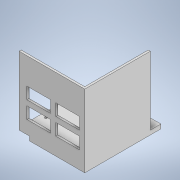
# Autodesk Inventor part: QUarter1
Saved by Autodesk Inventor 2020.2 (Build 242310000, 310)
## iProperties
Created: 2020-01-16
Part Number: QUarter1
Material: Generic
Document SubType Name: Modeling
Designer: ColinP
Density: 1 g/cm^3
Appearance: Default
Author: ColinP
Autodesk Inventor part; units mm, degrees
ref_plane "YZ Plane" through (0, 0, 0) normal (1, 0, 0) x (0, 1, 0)
ref_plane "XZ Plane" through (0, 0, 0) normal (0, 1, 0) x (-1, 0, 0)
ref_plane "XY Plane" through (0, 0, 0) normal (0, 0, 1) x (1, 0, 0)
sketch "Sketch3" plane through (0, 0, 0) normal (0, 1, 0) x (-1, 0, 0)
  line L0 (0, 0) -> (125, 0)
  line L1 (125, 0) -> (125, 125)
  line L2 (125, 125) -> (0, 125)
  line L3 (0, 125) -> (0, 0)
  dimension "d10" = 125
  dimension "d11" = 125
  constraints: 8 end point, 2 parallel, 1 horizontal, 1 perpendicular
  measures "d10" distance of L2.end L1.end
  measures "d11" distance of L1.end L0.end
extrude "Extrusion3" add sketch "Sketch3" along normal blind 10
sketch "Sketch8" plane through (0, 10, 0) normal (0, 1, 0) x (1, 0, 0)
  line L0 (0, 0) -> (-125, 0) projected
  line L1 (0, 0) -> (-4, 0)
  line L2 (-4, 0) -> (-4, -121)
  line L3 (-125, -125) -> (0, -125) projected
  line L4 (-4, -121) -> (-125, -121)
  line L5 (-125, 0) -> (-125, -125) projected
  line L6 (0, 0) -> (-125, 0) projected
  line L7 (-125, 0) -> (-125, -125) projected
  line L8 (-125, -125) -> (0, -125) projected
  line L9 (0, -125) -> (0, 0) projected
  dimension "d38" = 4
  dimension "d39" = 121
  dimension "d40" = 90
  constraints: 6 end point, 2 point on line, 1 perpendicular
  measures "d38" distance of L0.start L1.end
  measures "d39" distance of L1.end L2.end
  measures "d40" angle of L2 L4
extrude "Extrusion8" add sketch "Sketch8" along normal blind 125 contours L9 L3 L5 L4 L2 L0
sketch "Sketch9" plane through (-125, 0, 125) normal (0, 0, 1) x (1, 0, 0)
  line L0 (0, 0) -> (0, 10) projected
  line L1 (0, 10) -> (0, 30)
  line L2 (0, 0) -> (0, 135) projected
  line L3 (0, 30) -> (15, 30)
  line L4 (15, 30) -> (60, 30)
  line L5 (60, 30) -> (60, 52.5)
  line L6 (60, 52.5) -> (15, 52.5)
  line L7 (15, 52.5) -> (15, 30)
  line L8 (15, 52.5) -> (15, 62.5)
  line L9 (15, 62.5) -> (15, 85)
  line L10 (15, 85) -> (60, 85)
  line L11 (60, 85) -> (60, 62.5)
  line L12 (60, 62.5) -> (15, 62.5)
  line L13 (60, 62.5) -> (70, 62.5)
  line L14 (70, 62.5) -> (70, 85)
  line L15 (70, 85) -> (115, 85)
  line L16 (115, 85) -> (115, 62.5)
  line L17 (115, 62.5) -> (70, 62.5)
  line L18 (70, 52.5) -> (70, 62.5)
  line L19 (70, 52.5) -> (70, 30)
  line L20 (70, 30) -> (115, 30)
  line L21 (115, 30) -> (115, 52.5)
  line L22 (115, 52.5) -> (70, 52.5)
  point P0 (125, 0)
  dimension "d43" = 20
  dimension "d44" = 15
  dimension "d45" = 90
  dimension "d46" = 45
  dimension "d47" = 22.5
  dimension "d48" = 10
  dimension "d49" = 22.5
  dimension "d50" = 45
  dimension "d51" = 10
  dimension "d52" = 45
  dimension "d53" = 10
  dimension "d54" = 22.5
  dimension "d55" = 45
  constraints: 42 end point, 11 perpendicular, 11 point on line, 1 horizontal, 1 vertical
  measures "d43" distance of L0.end L1.end
  measures "d44" distance of L1.end L3.end
  measures "d45" angle of L1 L3
  measures "d46" distance of L3.end L4.end
  measures "d47" distance of L4.end L5.end
  measures "d48" distance of L6.end L8.end
  measures "d49" distance of L8.end L9.end
  measures "d50" distance of L9.end L10.end
  measures "d51" distance of L11.end L13.end
  measures "d52" distance of L14.end L15.end
  measures "d53" distance of L18.start L13.end
  measures "d54" distance of L18.start L19.end
  measures "d55" distance of L19.end L20.end
extrude "Extrusion9" cut sketch "Sketch9" against normal blind 10
sketch "Sketch10" plane through (-125, 0, 0) normal (-1, 0, 0) x (0, 0, 1)
  line L0 (0, 0) -> (125, 0)
  line L1 (125, 0) -> (125, 5)
  line L2 (0, 5) -> (0, 0)
  line L3 (125, 0) -> (125, 135) projected
  line L4 (125, 5) -> (10, 5)
  line L5 (10, 5) -> (10, 0)
  line L6 (0, 0) -> (125, 0) projected
  dimension "d59" = 5
  dimension "d62" = 125
  dimension "d63" = 115
  constraints: 10 end point, 2 horizontal, 2 perpendicular, 1 parallel, 1 point on line
  measures "d59" distance of L1.end L0.end
  measures "d62" distance of L2.start L1.end
  measures "d63" distance of L1.end L4.end
extrude "Extrusion12" cut sketch "Sketch10" against normal blind 20
sketch "Sketch13" plane through (0, 10, 0) normal (0, 1, 0) x (1, 0, 0)
  line L0 (-125, -10) -> (-105, -10) projected
  line L1 (-125, -10) -> (-125, -47)
  line L2 (-4, -121) -> (-125, -121) projected
  line L3 (-125, -47) -> (-115, -47)
  line L4 (-115, -47) -> (-115, -84)
  point P0 (0, 0)
  dimension "d79" = 37
  dimension "d80" = 10
  dimension "d81" = 37
  constraints: 6 end point, 3 perpendicular
  measures "d79" distance of L0.start L1.end
  measures "d80" distance of L1.end L3.end
  measures "d81" distance of L3.end L4.end
hole "Hole2" at (-115, 10, 84) at (-115, 10, 47) direction (0, -1, 0) diameter 4.318 end through all
sketch "Sketch14" plane through (0, 0, 0) normal (0, 0, -1) x (-1, 0, 0)
  line L0 (105, 0) -> (0, 0) projected
  line L1 (0, 0) -> (115, 0)
  line L2 (115, 0) -> (115, 5)
  line L3 (117.159, 5) -> (112.841, 5) projected
  line L4 (115, 5) -> (0, 5)
  line L5 (0, 0) -> (0, 135) projected
  line L6 (0, 0) -> (0, 5)
  dimension "d96" = 115
  dimension "d97" = 5
  constraints: 8 end point, 1 collinear, 1 horizontal, 1 midpoint, 1 perpendicular, 1 point on line
  measures "d96" distance of L0.end L1.end
  measures "d97" distance of L1.end L2.end
extrude "Extrusion14" add sketch "Sketch14" along normal blind 20
sketch "Sketch15" plane through (0, 10, 0) normal (0, 1, 0) x (1, 0, 0)
  line L0 (-115, 0) -> (-125, 0) projected
  line L1 (-115, 0) -> (-78, 0)
  line L2 (0, 0) -> (-115, 0) projected
  line L3 (-78, 0) -> (-78, 10)
  line L4 (-78, 10) -> (-41, 10)
  dimension "d100" = 37
  dimension "d101" = 10
  dimension "d102" = 37
  constraints: 6 end point, 2 perpendicular, 1 point on line
  measures "d100" distance of L0.start L1.end
  measures "d101" distance of L1.end L3.end
  measures "d102" distance of L3.end L4.end
hole "Hole3" at (-41, 10, -10) at (-78, 10, -10) direction (0, -1, 0) diameter 3.5 end through all
sketch "Sketch16" plane through (0, 0, 0) normal (0, -1, 0) x (1, 0, 0)
  line L0 (0, 0) -> (-115, 0) projected
  circle A0 centre (-41, -10) radius 1.75 projected
  circle A1 centre (-78, -10) radius 1.75 projected
  line L1 (-105, 10) -> (-125, 10) projected
  line L2 (-125, 0) -> (-125, 10) projected
  line L3 (-115, 0) -> (-125, 0) projected
  line L4 (-115, 0) -> (-115, -20) projected
  line L5 (0, -20) -> (-115, -20) projected
  line L6 (0, 125) -> (0, -20) projected
  line L7 (-105, 125) -> (0, 125) projected
  line L8 (-105, 125) -> (-105, 10) projected
extrude "Extrusion15" add sketch "Sketch16" along normal blind 3
sketch "Sketch17" plane through (0, -3, 0) normal (0, -1, 0) x (1, 0, 0)
  circle A0 centre (-41, -10) radius 1.75 projected
  circle A1 centre (-78, -10) radius 1.75 projected
  point P0 (0, 0)
hole "Hole4" at (-78, -3, -10) at (-41, -3, -10) direction (0, 1, 0) diameter 4.318 end through all counterbore diameter 7.62 counterbore depth 5.08
body "Solid2"
